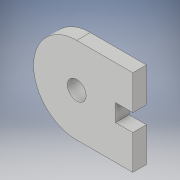
# Autodesk Inventor part: fakebattergasket2
Saved by Autodesk Inventor 2018.3 (Build 223284000, 284)
## iProperties
Created: 2019-09-05
Part Number: fakebattergasket2
Material: Generic
Document SubType Name: Modeling
Designer: Srinity
Density: 1 g/cm^3
Appearance: Default
Author: Srinity
Autodesk Inventor part; units mm, degrees
ref_plane "YZ Plane" through (0, 0, 0) normal (1, 0, 0) x (0, 1, 0)
ref_plane "XZ Plane" through (0, 0, 0) normal (0, 1, 0) x (-1, 0, 0)
ref_plane "XY Plane" through (0, 0, 0) normal (0, 0, 1) x (1, 0, 0)
sketch "Sketch1" plane through (0, 0, 0) normal (0, 0, 1) x (1, 0, 0)
  circle A0 centre (0, 0) radius 12.7
  line L0 (0, 12.7) -> (16.51, 12.7)
  line L1 (16.51, 12.7) -> (16.51, -12.7)
  line L2 (16.51, -12.7) -> (0, -12.7)
  line L3 (0, -12.7) -> (0, 12.7)
  dimension "d0" = 25.4
  dimension "d1" = 16.51
  constraints: 8 end point, 2 parallel, 2 tangent, 1 centre point, 1 coincident, 1 horizontal, 1 midpoint, 1 perpendicular
  measures "d0" diameter of A0
  measures "d1" distance of L0.start L0.end
extrude "Extrusion1" add sketch "Sketch1" along normal blind 4
sketch "Sketch2" plane through (16.51, -12.7, 0) normal (1, 0, 0) x (0, 0, -1)
  line L0 (-6.8327, 15.24) -> (9.0823, 15.24)
  line L1 (9.0823, 15.24) -> (9.0823, 10.16)
  line L2 (9.0823, 10.16) -> (-6.8327, 10.16)
  line L3 (-6.8327, 10.16) -> (-6.8327, 15.24)
  line L4 (0, 25.4) -> (0, 0) projected
  point P0 (0, 12.7)
  point P1 (9.0823, 12.7)
  point P2 (0, 12.7)
  dimension "d4" = 5.08
  constraints: 8 end point, 2 midpoint, 2 parallel, 1 horizontal, 1 horizontal alignment, 1 perpendicular
  measures "d4" distance of L0.end L1.end
extrude "Extrusion2" cut sketch "Sketch2" against normal blind 5.08
sketch "Sketch3" plane through (0, 0, 4) normal (0, 0, 1) x (1, 0, 0)
  circle A0 centre (0, 0) radius 2.75
  dimension "d7" = 5.5
  constraints: 1 centre point, 1 coincident
  measures "d7" diameter of A0
extrude "Extrusion3" cut sketch "Sketch3" against normal blind 7.62
body "Solid1"
